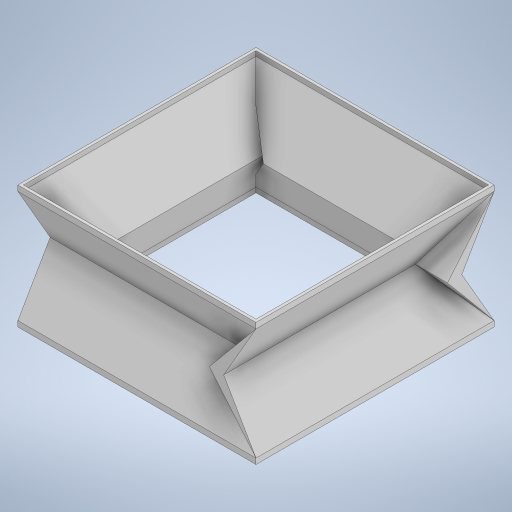
# Autodesk Inventor part: OV-PAM_n_4_standard_1F
Saved by Autodesk Inventor 2024 (Build 280153000, 153)
## iProperties
Created: 2023-08-31
Part Number: OV-PAM_n_4_standard_1F
Material: 일반
Document SubType Name: Modeling
Designer: jsw
Density: 1 g/cm^3
Appearance: 기본값
Author: jsw
Autodesk Inventor part; units mm, degrees
ref_plane "YZ Plane" through (0, 0, 0) normal (1, 0, 0) x (0, 1, 0)
sketch "스케치1" plane through (0, 0, 0) normal (0, 1, 0) x (-1, 0, 0)
  line L0 (-24.9446, 24.9446) -> (24.9446, 24.9446)
  line L1 (24.9446, 24.9446) -> (24.9446, -24.9446)
  line L2 (24.9446, -24.9446) -> (-24.9446, -24.9446)
  line L3 (-24.9446, -24.9446) -> (-24.9446, 24.9446)
  line L4 (-24.9446, 24.9446) -> (24.9446, -24.9446) construction
  line L5 (24.9446, 24.9446) -> (-24.9446, -24.9446) construction
  line L6 (-25.5446, 25.5446) -> (25.5446, 25.5446)
  line L7 (25.5446, 25.5446) -> (25.5446, -25.5446)
  line L8 (25.5446, -25.5446) -> (-25.5446, -25.5446)
  line L9 (-25.5446, -25.5446) -> (-25.5446, 25.5446)
  line L10 (-25.5446, 25.5446) -> (25.5446, -25.5446) construction
  line L11 (25.5446, 25.5446) -> (-25.5446, -25.5446) construction
  point P0 (0, 0)
  dimension "d0" = 70.554
  dimension "d1" = 0.6
  constraints: 24 end point, 4 midpoint, 4 parallel, 4 perpendicular, 2 horizontal
  measures "d0" distance of L0.start L1.end
  measures "d1" distance between parallel lines of L1 L7
extrude "돌출1" add sketch "스케치1" along normal blind 12 contours L0 L1 L2 L3 | L6 L7 L8 L9
ref_plane "작업 평면1" through (25.5446, 0, 25.5446) normal (-0.8660254, -0.5, 0) x (0, 0, -1)
sketch "스케치2" plane through (25.5446, 0, 25.5446) normal (1, 0, 0) x (0, 0, -1)
  line L0 (0, 0) -> (51.0892, 0) projected
  line L1 (51.0892, 0) -> (51.0892, 12) projected
  line L2 (0, 12) -> (51.0892, 12) projected
  line L3 (0, 0) -> (0, 12) projected
  line L4 (0, 0) -> (-14.301, 12)
  line L5 (-14.301, 12) -> (0, 12)
  line L6 (51.0892, 0) -> (41.0892, 12)
  point P0 (25.5446, 0)
  dimension "d5" = 140
  dimension "d6" = 10
  constraints: 6 end point, 1 collinear, 1 point on line
  measures "d5" angle of L4 L0
  measures "d6" distance of L6.end L1.end
extrude "돌출2" cut sketch "스케치2" against normal up to surface contours L3 L2 L6 L0 | L4 L5 L3 surface through (25.5446, 0, 25.5446) normal (-0.8660254, -0.5, 0)
pattern_circular "원형 패턴1" count 4 over 360 about axis through (0, -10, 0) along (0, 1, 0) of "돌출2"
ref_plane "작업 평면2" through (0, 12, 0) normal (0, 1, 0) x (1, 0, 0)
sketch "스케치3" plane through (0, 0, 0) normal (0, -1, 0) x (1, 0, 0)
  line L0 (25.5446, -25.5446) -> (-25.5446, -25.5446) projected
  line L1 (25.5446, 25.5446) -> (25.5446, -25.5446) projected
  line L2 (-25.5446, 25.5446) -> (25.5446, 25.5446) projected
  line L3 (-25.5446, -25.5446) -> (-25.5446, 25.5446) projected
  point P0 (0, 0)
extrude "돌출3" add sketch "스케치3" along normal blind 1.2
mirror "미러1" about plane through (0, 12, 0) normal (0, 1, 0) of "돌출2", "원형 패턴1", "돌출3", "돌출1"
shell "쉘1" thickness 0.6 removed faces 2 at (-8.5149, 25.2, 8.5149) at (-8.5149, -1.2, 8.5149)
